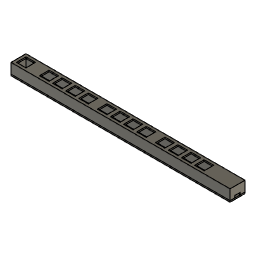
Fkeyboard (Autodesk Fusion 360 design; units mm, degrees)
Autodesk Fusion 360 part; units mm, degrees
sketch "Sketch1" plane through (0, 0, 0) normal (0, 0, 1) x (1, 0, 0)
  line L0 (-4, -4) -> (317.4, -4)
  line L1 (317.4, -4) -> (317.4, 17.9)
  line L2 (-4, 17.9) -> (-4, -4)
  line L3 (0, 0) -> (13.9, 0)
  line L4 (13.9, 0) -> (13.9, 13.9)
  line L5 (13.9, 13.9) -> (0, 13.9)
  line L6 (0, 13.9) -> (0, 0)
  line L7 (-2, -2) -> (315.4, -2)
  line L8 (315.4, -2) -> (315.4, 15.9)
  line L9 (-2, 15.9) -> (-2, -2)
  line L10 (-2, 15.9) -> (315.4, 15.9)
  line L11 (317.4, 17.9) -> (-4, 17.9)
  line L12 (-2, 6.95) -> (315.4, 6.95) construction
  line L13 (315.4, 6.95) -> (317.4, 6.95) construction
  line L14 (-2, 6.95) -> (-4, 6.95) construction
  line L15 (33.9, 13.9) -> (47.8, 13.9)
  line L16 (47.8, 13.9) -> (47.8, 0)
  line L17 (47.8, 0) -> (33.9, 0)
  line L18 (33.9, 0) -> (33.9, 13.9)
  line L19 (53.1, 13.9) -> (67, 13.9)
  line L20 (53.1, 0) -> (53.1, 13.9)
  line L21 (67, 13.9) -> (67, 0)
  line L22 (67, 0) -> (53.1, 0)
  line L23 (72.3, 13.9) -> (86.2, 13.9)
  line L24 (72.3, 0) -> (72.3, 13.9)
  line L25 (86.2, 13.9) -> (86.2, 0)
  line L26 (86.2, 0) -> (72.3, 0)
  line L27 (91.5, 13.9) -> (105.4, 13.9)
  line L28 (91.5, 0) -> (91.5, 13.9)
  line L29 (105.4, 13.9) -> (105.4, 0)
  line L30 (105.4, 0) -> (91.5, 0)
  line L31 (152, 0) -> (138.1, 0)
  line L32 (190.4, 13.9) -> (190.4, 0)
  line L33 (171.2, 13.9) -> (171.2, 0)
  line L34 (132.8, 13.9) -> (132.8, 0)
  line L35 (157.3, 13.9) -> (171.2, 13.9)
  line L36 (132.8, 0) -> (118.9, 0)
  line L37 (138.1, 0) -> (138.1, 13.9)
  line L38 (118.9, 0) -> (118.9, 13.9)
  line L39 (152, 13.9) -> (152, 0)
  line L40 (176.5, 13.9) -> (190.4, 13.9)
  line L41 (190.4, 0) -> (176.5, 0)
  line L42 (118.9, 13.9) -> (132.8, 13.9)
  line L43 (171.2, 0) -> (157.3, 0)
  line L44 (138.1, 13.9) -> (152, 13.9)
  line L45 (176.5, 0) -> (176.5, 13.9)
  line L46 (157.3, 0) -> (157.3, 13.9)
  line L47 (237, 0) -> (223.1, 0)
  line L48 (275.4, 13.9) -> (275.4, 0)
  line L49 (256.2, 13.9) -> (256.2, 0)
  line L50 (217.8, 13.9) -> (217.8, 0)
  line L51 (242.3, 13.9) -> (256.2, 13.9)
  line L52 (217.8, 0) -> (203.9, 0)
  line L53 (223.1, 0) -> (223.1, 13.9)
  line L54 (203.9, 0) -> (203.9, 13.9)
  line L55 (237, 13.9) -> (237, 0)
  line L56 (261.5, 13.9) -> (275.4, 13.9)
  line L57 (275.4, 0) -> (261.5, 0)
  line L58 (203.9, 13.9) -> (217.8, 13.9)
  line L59 (256.2, 0) -> (242.3, 0)
  line L60 (223.1, 13.9) -> (237, 13.9)
  line L61 (261.5, 0) -> (261.5, 13.9)
  line L62 (242.3, 0) -> (242.3, 13.9)
  line L63 (13.9, 0) -> (13.9, -2) construction
  line L64 (13.9, 13.9) -> (13.9, 15.9) construction
  line L65 (275.4, 13.9) -> (315.4, 13.9) construction
  circle A0 centre (23.9, 6.95) radius 1.5
  circle A1 centre (112.15, 6.95) radius 1.5
  circle A2 centre (197.15, 6.95) radius 1.5
  line L66 (13.9, 0) -> (33.9, 13.9) construction
  line L67 (105.4, 0) -> (118.9, 13.9) construction
  line L68 (190.4, 0) -> (203.9, 13.9) construction
  circle A3 centre (23.9, 6.95) radius 2.5
  circle A4 centre (112.15, 6.95) radius 2.5
  circle A5 centre (197.15, 6.95) radius 2.5
  line L69 (315.4, 15.95) -> (282.4, 15.95) construction
  line L70 (282.4, 15.95) -> (282.4, -2.05) construction
  line L71 (282.4, -2.05) -> (315.4, -2.05) construction
  line L72 (315.4, -2.05) -> (315.4, 15.95) construction
  circle A6 centre (278.9, 6.95) radius 1.5
  circle A7 centre (278.9, 6.95) radius 2.5
  line L73 (282.4, 13.9) -> (275.4, 0) construction
  dimension "d1" = 13.9
  dimension "d6" = 4
  dimension "d7" = 4
  dimension "d12" = 2
  dimension "d13" = 2
  dimension "d33" = 20
  dimension "d36" = 19.2
  dimension "d37" = 0
  dimension "d40" = 85
  dimension "d41" = 0
  dimension "d42" = 40
  dimension "d43" = 33
  dimension "d44" = 18
  dimension "d45" = 3
  dimension "d46" = 5
  constraint horizontal L0
  constraint horizontal L3
  constraint vertical L4
  constraint horizontal L5
  constraint vertical L6
  constraint coincident L3.start L6.end
  constraint equal L3 L6
  constraint horizontal L7
  constraint perpendicular L8 L10
  constraint perpendicular L2 L11
  constraint midpoint L9 L12.start
  constraint midpoint L8 L12.end
  constraint midpoint L1 L13.end
  constraint horizontal L13
  constraint midpoint L2 L14.end
  constraint perpendicular L2 L14
  constraint equal L13 L14
  constraint vertical L1
  constraint horizontal L15
  constraint vertical L16
  constraint horizontal L17
  constraint vertical L18
  constraint equal L3 L17
  constraint equal L6 L18
  constraint collinear L5 L15
  constraint coincident L7 L63.end
  constraint perpendicular L7 L63
  constraint coincident L10 L64.end
  constraint perpendicular L10 L64
  constraint equal L63 L64
  constraint coincident L8 L65.end
  constraint perpendicular L8 L65
  constraint coincident L12 A0.centre
  constraint coincident L12 A1.centre
  constraint coincident L12 A2.centre
  constraint equal A0 A1
  constraint equal A1 A2
  constraint coincident A2.centre L68
  constraint coincident A1.centre L67
  constraint coincident A0.centre L66
  constraint concentric A0 A3
  constraint concentric A1 A4
  constraint concentric A2 A5
  constraint horizontal L69
  constraint vertical L70
  constraint horizontal L71
  constraint vertical L72
  constraint collinear L8 L72
  constraint symmetric L12 L69 L71
  constraint coincident L12 A6.centre
  constraint concentric A6 A7
  constraint equal A2 A6
  constraint equal A5 A7
  constraint equal A4 A5
  constraint equal A3 A4
  constraint coincident L70 L73.start
  constraint coincident L65 L73.start
  constraint coincident A6.centre L73
  measures "d1" distance of L3.start L3.end
  measures "d6" distance of L2 L6
  measures "d7" distance of L0 L3
  measures "d12" distance of L2 L9
  measures "d13" distance of L0 L7.start
  measures "d33" distance of L4 L18
  measures "d42" distance of L48.start L65.end
  measures "d43" distance of L69.start L69.end
  measures "d44" distance of L69.end L70.end
  measures "d45" diameter of A0
  measures "d46" diameter of A3
extrude "Extrude1" add sketch "Sketch1" along normal blind 2 contours L0 L1 L2 L11 | L7 L8 L9 L10 | A0 | A1 | A2 | A3 | A4 | A5 | A6 | A7 makes body 1
extrude "Extrude2" add sketch "Sketch1" against normal blind 13 contours L0 L1 L2 L11 bodies 1
extrude "Extrude3" add sketch "Sketch1" against normal up to surface (13 mm away) contours A3 | A4 | A5 | A7 bodies 1
sketch "Sketch2" plane through (317.4, 0, 0) normal (1, 0, 0) x (0, 1, 0)
  line L0 (-315.4, 0) -> (-315.4, -13)
  line L1 (2.95, -13) -> (10.95, -13)
  line L2 (10.95, -13) -> (10.95, -10)
  line L3 (10.95, -10) -> (2.95, -10)
  line L4 (2.95, -10) -> (2.95, -13)
  line L5 (6.95, -5.5) -> (6.95, -10) construction
  line L6 (17.9, -13) -> (-4, -13)
  line L7 (17.9, 2) -> (17.9, -13)
  line L8 (-4, -13) -> (-4, 2)
  point P0 (-317.4, -13)
  dimension "d22" = 8
  dimension "d23" = 3
  constraint horizontal L1
  constraint vertical L2
  constraint horizontal L3
  constraint vertical L4
  constraint midpoint L3 L5.end
  constraint vertical L5
  constraint collinear L1 L6
  measures "d22" distance of L1.start L1.end
  measures "d23" distance of L1.end L2.end
extrude "Extrude4" cut sketch "Sketch2" against normal blind 5 bodies 1
sketch "Sketch1 (2)" plane through (0, 0, -13) normal (0, 0, -1) x (1, 0, 0) in component "Component"
  line L0 (-4, 4) -> (317.4, 4)
  line L1 (317.4, 4) -> (317.4, -17.9)
  line L2 (317.4, -17.9) -> (-4, -17.9)
  line L3 (-4, -17.9) -> (-4, 4)
  line L4 (-4, -17.9) -> (317.4, -17.9)
  line L5 (-4, 4) -> (-4, -17.9)
  circle A0 centre (23.9, -6.95) radius 1.5
  circle A1 centre (112.15, -6.95) radius 1.5
  circle A2 centre (197.15, -6.95) radius 1.5
  circle A3 centre (278.9, -6.95) radius 1.5
  circle A4 centre (23.9, -6.95) radius 1.5
  circle A5 centre (112.15, -6.95) radius 1.5
  circle A6 centre (197.15, -6.95) radius 1.5
  circle A7 centre (278.9, -6.95) radius 1.5
  constraint horizontal L0
  constraint vertical L1
  constraint horizontal L2
  constraint vertical L3
  constraint coincident L1.end L4
  constraint coincident L1 L2.start
  constraint coincident L0.start L5
  constraint coincident L0 L3.end
  constraint equal A2 A3
  constraint equal A1 A2
  constraint equal A0 A1
  constraint concentric A0 A4
  constraint concentric A1 A5
  constraint concentric A2 A6
  constraint concentric A3 A7
  constraint equal A3 A7
extrude "Extrude1'" add sketch "Sketch1 (2)" along normal blind 2 separate body makes body 2 in component "Component"
chamfer "Chaflán1" distance 2 angle 45 4 edges at (22.5015, 6.4076, -15) (110.7515, 6.4076, -15) (195.7515, 6.4076, -15) (277.5015, 6.4076, -15) on bodies 2 in component "Component"
component "Component" placed x (1, 0, 0) y (0, 1, 0) z (0, 0, 1) at (0, 0, 0)
equation "d6 = d7"
equation "d36 = 13.9 mm + 5.3 mm"
